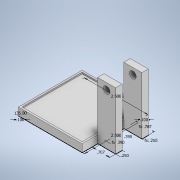
# Autodesk Inventor part: wastebottleholder
Saved by Autodesk Inventor 2020 (Build 240168000, 168)
## iProperties
Created: 2020-02-07
Part Number: wastebottleholder
Material: Generic
Document SubType Name: Modeling
Designer: pab2
Density: 1 g/cm^3
Appearance: Default
Author: pab2
Autodesk Inventor part; units mm, degrees
ref_plane "YZ Plane" through (0, 0, 0) normal (1, 0, 0) x (0, 1, 0)
ref_plane "XZ Plane" through (0, 0, 0) normal (0, 1, 0) x (-1, 0, 0)
ref_plane "XY Plane" through (0, 0, 0) normal (0, 0, 1) x (1, 0, 0)
sketch "Sketch1" plane through (0, 0, 0) normal (0, 1, 0) x (-1, 0, 0)
  line L0 (0, 0) -> (-63.5, 0)
  line L1 (-63.5, 0) -> (-63.5, -63.5)
  line L2 (-63.5, -63.5) -> (0, -63.5)
  line L3 (0, -63.5) -> (0, 0)
  line L4 (-63.5, -57.15) -> (-63.5, -63.5)
  line L5 (-63.5, -6.35) -> (-63.5, 0)
  line L6 (-63.5, -31.75) -> (-63.5, -41.656)
  line L7 (-63.5, -31.75) -> (-63.5, -21.844)
  line L8 (-63.5, -21.844) -> (-81.4578, -21.844)
  line L9 (-81.4578, -21.844) -> (-81.4578, -15.494)
  line L10 (-81.4578, -15.494) -> (-63.5, -15.494)
  line L11 (-63.5, -15.494) -> (-63.5, -21.844)
  line L12 (-63.5, -41.656) -> (-81.4578, -41.656)
  line L13 (-81.4578, -41.656) -> (-81.4578, -48.006)
  line L14 (-81.4578, -48.006) -> (-63.5, -48.006)
  line L15 (-63.5, -48.006) -> (-63.5, -41.656)
  line L16 (0, 0) -> (-1.7961, -1.7961)
  line L17 (0, 0) -> (2.54, 0) construction
  line L18 (-63.5, -63.5) -> (-61.7039, -61.7039)
  line L19 (-1.7961, -1.7961) -> (-61.7039, -1.7961)
  line L20 (-61.7039, -1.7961) -> (-61.7039, -61.7039)
  line L21 (-61.7039, -61.7039) -> (-1.7961, -61.7039)
  line L22 (-1.7961, -61.7039) -> (-1.7961, -1.7961)
  point P0 (-63.5, -15.494)
  dimension "PlatformL" = 63.5
  dimension "PlatformW" = 63.5
  dimension "SideThickness" = 9.906
  dimension "d12" = 9.906
  dimension "EarWidth" = 17.9578
  dimension "EarThickness" = 6.35
  dimension "d15" = 17.9578
  dimension "d16" = 6.35
  dimension "d26" = 2.54
  dimension "d27" = 135
  dimension "d28" = 2.54
  constraints: 46 end point, 8 parallel, 5 horizontal, 4 perpendicular, 2 point on line, 1 equal length, 1 midpoint
  measures "PlatformL" distance of L2.end L1.end
  measures "PlatformW" distance of L1.end L0.end
  measures "SideThickness" distance of L6.start L6.end
  measures "d12" distance of L6.start L7.end
  measures "EarWidth" distance of L9.end L10.end
  measures "EarThickness" distance of L8.end L9.end
  measures "d15" distance of L14.end L13.end
  measures "d16" distance of L13.end L12.end
  measures "d26" distance of L0.start L16.end
  measures "d27" angle of L16 L17
  measures "d28" distance of L1.end L18.end
extrude "Extrusion1" add sketch "Sketch1" along normal blind 6.35 contours L22 L21 L20 L19
extrude "Extrusion2" add sketch "Sketch1" along normal blind 57.15 contours L1 L8 L9 L10 | L14 L13 L12 L1
sketch "Sketch3" plane through (63.5, 0, -15.494) normal (0, 0, 1) x (1, 0, 0)
  line L0 (0, 0) -> (17.9578, 0) projected
  line L1 (8.9789, 0) -> (8.9789, 50.8)
  line L2 (8.9789, 0) -> (59.7789, 0) construction
  point P0 (-63.5, 0)
  dimension "HeightToHole" = 50.8
  dimension "d18" = 90
  constraints: 4 end point, 1 horizontal, 1 midpoint, 1 perpendicular, 1 vertical
  measures "HeightToHole" distance of L1.start L1.end
  measures "d18" angle of L2 L1
hole "Hole1" at (72.4789, 50.8, -15.494) direction (0, 0, -1) diameter 6.7564 end through all clearance for "Flat Head Machine Screw (82)" size "1/4" standard "Ansi Unified Screw Threads"
extrude "Extrusion3" add sketch "Sketch1" along normal blind 7.62 contours L16 L19 L20 L18 L1 L0 | L3 L2 L18 L21 L22 L16
equation "\"d12\" = SideThickness"
equation "\"d15\" = EarWidth"
equation "\"d16\" = EarThickness"
body "Solid1"
